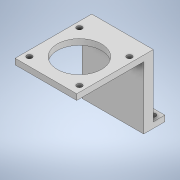
# Autodesk Inventor part: Motor_Mount
Saved by Autodesk Inventor 2022.3 (Build 263350000, 350)
## iProperties
Created: 2022-05-27
Part Number: Motor_Mount
Material: Generic
Document SubType Name: Modeling
Designer: Mlees
Density: 1 g/cm^3
Appearance: Default
Author: Mlees
Autodesk Inventor part; units mm, degrees
ref_plane "YZ Plane" through (0, 0, 0) normal (1, 0, 0) x (0, 1, 0)
ref_plane "XZ Plane" through (0, 0, 0) normal (0, 1, 0) x (-1, 0, 0)
ref_plane "XY Plane" through (0, 0, 0) normal (0, 0, 1) x (1, 0, 0)
sketch "Sketch1" plane through (0, 0, 0) normal (0, 1, 0) x (-1, 0, 0)
  line L0 (0, 0) -> (32, 0)
  line L1 (16, 0) -> (29, 0)
  circle A0 centre (29, 3) radius 1.375
  line L2 (16, 0) -> (16, 4.375)
  circle A1 centre (3, 3) radius 1.375
  line L3 (0, 0) -> (0, 6)
  line L4 (0, 6) -> (0, 11)
  line L5 (0, 11) -> (32, 11)
  line L6 (32, 11) -> (32, 0)
  dimension "d3" = 2.75
  dimension "d4" = 6
  dimension "d5" = 5
  constraints: 14 end point, 2 centre point, 2 perpendicular, 2 point on line, 2 vertical, 1 horizontal, 1 midpoint, 1 symmetric about line, 1 other
  measures "d3" diameter of A0
  measures "d4" distance of L0.start L3.end
  measures "d5" distance of L3.end L4.end
extrude "Extrusion1" add sketch "Sketch1" along normal blind 3
sketch "Sketch2" plane through (0, 3, 0) normal (0, 1, 0) x (1, 0, 0)
  line L0 (-32, -11) -> (0, -11) projected
  line L1 (0, -11) -> (0, 0) projected
  line L2 (-32, -11) -> (0, -11)
  line L3 (0, -11) -> (0, -6)
  line L4 (0, -6) -> (-32, -6)
  line L5 (-32, -6) -> (-32, -11)
  dimension "d8" = 5
  constraints: 8 end point, 2 parallel, 1 horizontal, 1 perpendicular, 1 point on line
  measures "d8" distance of L3.end L2.end
extrude "Extrusion2" add sketch "Sketch2" along normal blind 29.5
sketch "Sketch3" plane through (0, 32.5, 0) normal (0, 1, 0) x (1, 0, 0)
  circle A0 centre (-3, -3) radius 1.375 projected
  line L0 (-3, -3) -> (-3, -11)
  line L1 (-32, -11) -> (0, -11) projected
  line L2 (-3, -11) -> (-3, -15.4)
  circle A1 centre (-29, -3) radius 1.375 projected
  line L3 (-29, -3) -> (-29, -11)
  line L4 (-29, -11) -> (-29, -15.4)
  circle A2 centre (-29, -15.4) radius 1.375
  circle A3 centre (-3, -15.4) radius 1.375
  line L5 (-3, -15.4) -> (-3, -41.4)
  circle A4 centre (-3, -41.4) radius 1.375
  circle A5 centre (-29, -41.4) radius 1.375
  line L6 (0, -6) -> (-32, -6) projected
  line L7 (-32, -6) -> (0, -6)
  line L8 (0, -6) -> (0, -45.8)
  line L9 (0, -45.8) -> (-32, -45.8)
  line L10 (-32, -45.8) -> (-32, -6)
  point P0 (0, 0)
  dimension "d11" = 4.4
  dimension "d12" = 2.75
  dimension "d13" = 26
  dimension "d14" = 39.8
  constraints: 18 end point, 4 centre point, 4 point on line, 3 coincident, 2 parallel, 2 perpendicular, 2 vertical, 1 horizontal
  measures "d11" distance of L0.end L2.end
  measures "d12" diameter of A2
  measures "d13" distance of L5.start L5.end
  measures "d14" distance of L7.end L8.end
extrude "Extrusion3" add sketch "Sketch3" along normal blind 3 contours L6 L8 L1 L0 | L0 L1 L3 L6 | L1 L8 L9 L10 | L3 L1 L10 L6
sketch "Sketch4" plane through (0, 35.5, 0) normal (0, 1, 0) x (1, 0, 0)
  circle A0 centre (-3, -15.4) radius 1.375 projected
  circle A1 centre (-29, -41.4) radius 1.375 projected
  circle A2 centre (-29, -15.4) radius 1.375 projected
  circle A3 centre (-3, -41.4) radius 1.375 projected
  circle A4 centre (-16, -28.4) radius 11.5
  point P0 (0, 0)
  dimension "d17" = 23
  constraints: 1 centre point
  measures "d17" diameter of A4
extrude "Extrusion4" cut sketch "Sketch4" against normal blind 3 contours A4
body "Solid1"
